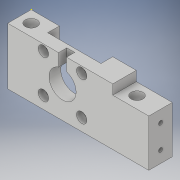
# Autodesk Inventor part: ps system back mount
Saved by Autodesk Inventor 2017 (Build 210142000, 142)
## iProperties
Created: 2016-07-18
Part Number: ps system back mount
Material: Generic
Document SubType Name: Modeling
Designer: Darien Morrow
Density: 1 g/cm^3
Appearance: Default
Author: Darien Morrow
Autodesk Inventor part; units mm, degrees
ref_plane "YZ Plane" through (0, 0, 0) normal (1, 0, 0) x (0, 1, 0)
ref_plane "XZ Plane" through (0, 0, 0) normal (0, 1, 0) x (-1, 0, 0)
ref_plane "XY Plane" through (0, 0, 0) normal (0, 0, 1) x (1, 0, 0)
sketch "Sketch1" plane through (0, 0, 0) normal (0, 0, 1) x (1, 0, 0)
  line L0 (0, 0) -> (114.3, 0)
  line L1 (114.3, 0) -> (114.3, 46.0375)
  line L2 (114.3, 46.0375) -> (0, 46.0375)
  line L3 (0, 46.0375) -> (0, 0)
  line L4 (69.85, 46.0375) -> (19.05, 46.0375)
  point P0 (44.45, 46.0375)
  dimension "d0" = 114.3
  dimension "d1" = 46.0375
  dimension "d62" = 69.85
  constraints: 10 end point, 2 horizontal, 2 parallel, 1 midpoint, 1 perpendicular, 1 point on line
  measures "d0" distance between parallel lines of L1 L3
  measures "d1" distance between parallel lines of L0 L2
  measures "d62" distance from line of point (44.45, 46.037) L1
extrude "Extrusion1" add sketch "Sketch1" along normal blind 19.05
sketch "Sketch2" plane through (0, 0, 0) normal (0, 0, -1) x (-1, 0, 0)
  line L0 (-114.3, 46.0375) -> (0, 46.0375) projected
  line L1 (-114.3, 0) -> (-114.3, 46.0375) projected
  point P0 (0, 0)
  point P1 (-44.45, 25.4)
  point P2 (-19.05, 38.1)
  point P3 (0, 46.0375)
  dimension "d7" = 20.6375
  dimension "d8" = 69.85
  constraints: 1 other
  measures "d8" distance from line of L1 point (-44.45, 25.4)
hole "Hole1" at (44.45, 25.4, 0) direction (0, 0, 1) diameter 22 depth 25.4 tip angle 118
sketch "Sketch3" plane through (0, 0, 0) normal (0, 0, -1) x (-1, 0, 0)
  line L0 (-66.04, 3.81) -> (-22.86, 3.81)
  line L1 (-22.86, 3.81) -> (-22.86, 46.99)
  line L2 (-22.86, 46.99) -> (-66.04, 46.99)
  line L3 (-66.04, 46.99) -> (-66.04, 3.81)
  line L4 (-66.04, 3.81) -> (-22.86, 46.99) construction
  line L5 (-22.86, 3.81) -> (-66.04, 46.99) construction
  line L6 (-114.3, 46.0375) -> (0, 46.0375) projected
  line L7 (-69.85, 46.0375) -> (-19.05, 46.0375) projected
  line L8 (-66.04, 46.99) -> (-22.86, 46.99)
  line L9 (-22.86, 46.99) -> (-22.86, 46.0375)
  line L10 (-22.86, 46.0375) -> (-66.04, 46.0375)
  line L11 (-66.04, 46.0375) -> (-66.04, 46.99)
  line L12 (-114.3, 0) -> (-114.3, 46.0375) projected
  point P0 (0, 0)
  point P1 (-44.45, 25.4)
  point P2 (-19.05, 38.1)
  point P3 (0, 46.0375)
  dimension "d16" = 20.6375
  dimension "d17" = 43.18
  dimension "d18" = 43.18
  dimension "d21" = 69.85
  dimension "d22" = 43.18
  constraints: 20 end point, 4 parallel, 2 horizontal, 2 midpoint, 2 perpendicular, 1 point on line, 1 other
  measures "d17" distance between parallel lines of L0 L2
  measures "d18" distance between parallel lines of L1 L3
  measures "d21" distance from line of point (-44.45, 25.4) L12
  measures "d22" distance between parallel lines of L9 L11
extrude "Extrusion2" cut sketch "Sketch3" against normal blind 9.525
sketch "Sketch4" plane through (0, 0, 19.05) normal (0, 0, 1) x (1, 0, 0)
  line L0 (28.95, 9.9) -> (59.95, 9.9)
  line L1 (59.95, 9.9) -> (59.95, 40.9)
  line L2 (59.95, 40.9) -> (28.95, 40.9)
  line L3 (28.95, 40.9) -> (28.95, 9.9)
  line L4 (28.95, 9.9) -> (59.95, 40.9) construction
  line L5 (59.95, 9.9) -> (28.95, 40.9) construction
  line L6 (114.3, 46.0375) -> (0, 46.0375) projected
  line L7 (114.3, 0) -> (114.3, 46.0375) projected
  point P0 (0, 0)
  point P1 (44.45, 25.4)
  point P2 (69.85, 38.1)
  point P3 (0, 46.0375)
  dimension "d23" = 20.6375
  dimension "d24" = 69.85
  dimension "d25" = 31
  dimension "d26" = 31
  constraints: 12 end point, 3 coincident, 2 midpoint, 2 parallel, 1 horizontal, 1 perpendicular, 1 other
  measures "d24" distance from line of L7 point (44.45, 25.4)
  measures "d25" distance between parallel lines of L1 L3
  measures "d26" distance between parallel lines of L0 L2
hole "Hole2" at (28.95, 40.9, 19.05) at (28.95, 9.9, 19.05) at (59.95, 40.9, 19.05) at (59.95, 9.9, 19.05) direction (0, 0, -1) diameter 3.4036 end through all counterbore diameter 8.4074 counterbore depth 5.715 clearance for "Hex Head Machine Screw" size "M3" standard "Ansi Metric M Profile"
sketch "Sketch5" plane through (0, 0, 0) normal (0, -1, 0) x (1, 0, 0)
  line L0 (95.25, 9.525) -> (9.525, 9.525)
  line L1 (0, 0) -> (114.3, 0) projected
  line L2 (114.3, 0) -> (114.3, 19.05) projected
  dimension "d34" = 85.725
  dimension "d35" = 9.525
  dimension "d36" = 19.05
  constraints: 2 coincident, 2 end point, 1 horizontal
  measures "d34" distance of L0.end L0.start
  measures "d35" distance between parallel lines of L0 L1
  measures "d36" distance from line of L0.start L2
hole "Hole3" at (95.25, 0, 9.525) at (9.525, 0, 9.525) direction (0, 1, 0) diameter 9.6012 end through all
sketch "Sketch6" plane through (0, 0, 0) normal (0, 0, -1) x (-1, 0, 0)
  line L0 (-114.3, 46.0375) -> (0, 46.0375) projected
  line L1 (0, 46.0375) -> (0, 0) projected
  line L2 (0, 0) -> (-114.3, 0) projected
  line L3 (-100.0506, 46.0375) -> (-90.4494, 46.0375) projected
  line L4 (-114.3, 0) -> (-114.3, 46.0375) projected
  line L5 (-14.3256, 46.0375) -> (-4.7244, 46.0375) projected
  point P0 (-19.05, 38.1)
  point P1 (-95.25, 19.05)
  point P2 (-9.525, 19.05)
  point P3 (-19.05, 46.0375)
  point P4 (-22.86, 0)
  dimension "d105" = 19.05
  dimension "d108" = 19.05
  dimension "d110" = 9.6012
  dimension "d111" = 4.8006
  dimension "d112" = 9.525
  constraints: 1 other
  measures "d105" distance from line of L2 point (-9.525, 19.05)
  measures "d108" distance from line of L2 point (-95.25, 19.05)
  measures "d110" distance of L3.start L3.end
  measures "d111" horizontal distance of point (-95.25, 19.05) L3.end
  measures "d112" distance from line of L1 point (-9.525, 19.05)
hole "Hole4" at (95.25, 19.05, 0) at (9.525, 19.05, 0) direction (0, 0, 1) diameter 3.302 depth 12.2936 tip angle 118 thread size "8-32 UNC" class "2B" standard "ANSI Unified Screw Threads"
sketch "Sketch8" plane through (114.3, 0, 0) normal (1, 0, 0) x (0, 0, -1)
  line L0 (-19.05, 46.0375) -> (-19.05, 0) projected
  line L1 (0, 0) -> (-19.05, 0) projected
  line L2 (0, 46.0375) -> (-19.05, 46.0375) projected
  point P0 (-9.525, 9.525)
  point P1 (-9.525, 28.575)
  dimension "d87" = 19.05
  dimension "d88" = 9.525
  dimension "d90" = 9.525
  dimension "d99" = 9.525
  measures "d87" distance of point (-9.525, 28.575) point (-9.525, 9.525)
  measures "d88" distance from line of L0 point (-9.525, 9.525)
  measures "d90" distance from line of point (-9.525, 9.525) L1
  measures "d99" distance from line of L0 point (-9.525, 28.575)
hole "Hole8" at (114.3, 9.525, 9.525) at (114.3, 28.575, 9.525) direction (-1, 0, 0) diameter 3.302 depth 12.2936 tip angle 118 thread size "8-32 UNC" class "2B" standard "ANSI Unified Screw Threads"
sketch "Sketch11" plane through (0, 46.0375, 19.05) normal (0, 1, 0) x (1, 0, 0)
  line L0 (66.04, 9.525) -> (22.86, 9.525) projected
  line L1 (114.3, 0) -> (0, 0) projected
  line L2 (22.86, 9.525) -> (22.86, 19.05) projected
  line L3 (66.04, 19.05) -> (66.04, 9.525) projected
  point P0 (0, 19.05)
  point P1 (44.45, 4.7625)
  dimension "d114" = 9.525
  dimension "d115" = 43.18
  dimension "d116" = 4.7625
  dimension "d117" = 21.59
  measures "d114" distance between parallel lines of L0 L1
  measures "d115" distance between parallel lines of L2 L3
  measures "d116" distance from line of L0 point (44.45, 4.763)
  measures "d117" distance from line of point (44.45, 4.763) L2
hole "Hole9" at (44.45, 46.0375, 14.2875) direction (0, -1, 0) diameter 3.81 depth 19.05 tip angle 118 clearance for "Hex Machine Screw" size "#6" standard "Ansi Unified Screw Threads"
sketch "Sketch14" plane through (0, 46.0375, 19.05) normal (0, 1, 0) x (1, 0, 0)
  line L0 (0, 0) -> (114.3, 0) projected
  line L1 (0, 19.05) -> (114.3, 19.05) projected
  line L2 (114.3, 0) -> (85.09, 0)
  line L3 (85.09, 0) -> (85.09, 19.05)
  line L4 (85.09, 19.05) -> (114.3, 19.05)
  line L5 (114.3, 19.05) -> (114.3, 0)
  dimension "d130" = 29.21
  constraints: 8 end point, 2 parallel, 1 horizontal, 1 perpendicular, 1 point on line
  measures "d130" distance of L3.end L4.end
extrude "Extrusion5" cut sketch "Sketch14" against normal blind 7.9375
sketch "Sketch15" plane through (0, 0, 0) normal (0, 0, -1) x (-1, 0, 0)
  line L0 (-22.86, 3.81) -> (-66.04, 3.81) projected
  line L1 (-66.04, 3.81) -> (-66.04, 46.0375) projected
  line L2 (-85.09, 38.1) -> (-114.3, 38.1) projected
  line L3 (-85.09, 46.0375) -> (-85.09, 38.1) projected
  point P0 (0, 0)
  point P1 (-78.74, 15.875)
  point P2 (-85.09, 33.782)
  dimension "d133" = 12.065
  dimension "d134" = 12.7
  dimension "d135" = 4.318
  dimension "d136" = 0
  measures "d133" distance from line of point (-78.74, 15.875) L0
  measures "d134" distance from line of point (-78.74, 15.875) L1
  measures "d135" distance from line of point (-85.09, 33.782) L2
  measures "d136" distance from line of point (-85.09, 33.782) L3
hole "Hole10" at (78.74, 15.875, 0) at (85.09, 33.782, 0) direction (0, 0, 1) diameter 3.302 depth 12.2936 tip angle 118 thread size "8-32 UNC" class "2B" standard "ANSI Unified Screw Threads"
sketch "Sketch16" plane through (0, 46.0375, 19.05) normal (0, 1, 0) x (1, 0, 0)
  point P0 (0, 19.05)
sketch "Sketch17" plane through (0, 46.0375, 19.05) normal (0, 1, 0) x (1, 0, 0)
  circle A0 centre (44.45, 4.7625) radius 1.905 projected
  line L0 (0, 0) -> (114.3, 0) projected
  line L1 (44.45, 6.6675) -> (41.2634, 6.6675)
  line L2 (41.2634, 6.6675) -> (41.2634, 0)
  line L3 (41.2634, 0) -> (44.45, 0)
  line L4 (44.45, 0) -> (44.45, 6.6675)
  line L5 (44.45, 6.6675) -> (47.625, 6.6675)
  line L6 (47.625, 6.6675) -> (47.625, 0)
  line L7 (47.625, 0) -> (44.45, 0)
  line L8 (44.45, 0) -> (44.45, 6.6675)
  point P0 (0, 19.05)
  dimension "d144" = 3.175
  constraints: 16 end point, 4 parallel, 2 horizontal, 2 perpendicular, 2 point on line, 1 vertical alignment, 1 other
  measures "d144" distance between parallel lines of L4 L6
extrude "Extrusion6" cut sketch "Sketch17" against normal blind 25.4
sketch "Sketch9" plane through (0, 0, 0) normal (0, 0, -1) x (-1, 0, 0)
  line L0 (-139.7, 41.275) -> (0, 41.275)
  line L1 (0, 0) -> (-114.3, 0) projected
  line L2 (-101.6, 31.369) -> (-38.1, 31.369)
  line L3 (0, 46.0375) -> (0, 0) projected
  line L4 (-19.05, 46.0375) -> (0, 46.0375) projected
  line L5 (0, 46.0375) -> (-31.75, 41.275)
  line L6 (-4.5219, 55.376) -> (-36.0166, 50.6518)
  point P0 (-19.05, 38.1)
  point P1 (-23.7267, 67.9523)
  dimension "d63" = 41.275
  dimension "d64" = 9.906
  dimension "d65" = 139.7
  dimension "d66" = 0
  dimension "d67" = 31.75
  dimension "d68" = 9.906
  dimension "d69" = 9.906
  dimension "d71" = 63.5
  dimension "d72" = 38.1
  constraints: 8 end point, 2 coincident, 2 horizontal, 1 point on line
  measures "d63" distance between parallel lines of L0 L1
  measures "d64" distance between parallel lines of L2 L0
  measures "d65" distance of L0.end L0.start
  measures "d66" distance from line of L0.end L3
  measures "d67" distance of L0.end L5.end
  measures "d68" distance from line of L5 L6.start
  measures "d69" distance from line of L5 L6.end
  measures "d71" distance of L2.end L2.start
  measures "d72" distance from line of L3 L2.end
sketch "Sketch7" plane through (0, 0, 0) normal (-1, 0, 0) x (0, 0, 1)
  line L0 (9.525, 46.0375) -> (9.525, 3.81) projected
  line L1 (9.525, 24.9237) -> (9.525, -32.2263)
  point P0 (0, 0)
  point P1 (9.525, 89.85)
  dimension "d54" = 57.15
  constraints: 2 coincident, 2 end point, 1 collinear, 1 midpoint
  measures "d54" distance of L1.end L1.start
equation "\"d108\" = d105"
body "Solid1"
